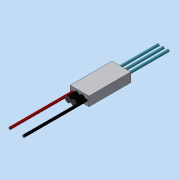
# Autodesk Inventor part: Turnigy_ESC
Saved by Autodesk Inventor 2015 SP1 (Build 190203100, 203)
## iProperties
Created: 2015-06-19
Part Number: Turnigy_ESC
Material: PPS Plastic
Document SubType Name: Modeling
Designer: YOUR_NAME_HERE
Density: 1.637 g/cm^3
Appearance: Smooth - White
Author: YOUR_NAME_HERE
Autodesk Inventor part; units mm, degrees
ref_plane "YZ Plane" through (0, 0, 0) normal (1, 0, 0) x (0, 1, 0)
ref_plane "XZ Plane" through (0, 0, 0) normal (0, 1, 0) x (-1, 0, 0)
ref_plane "XY Plane" through (0, 0, 0) normal (0, 0, 1) x (1, 0, 0)
sketch "Sketch1" plane through (0, 0, 0) normal (0, 1, 0) x (-1, 0, 0)
  line L0 (17, 38) -> (-17, 38)
  line L1 (-17, 38) -> (-17, -38)
  line L2 (-17, -38) -> (17, -38)
  line L3 (17, -38) -> (17, 38)
  line L4 (23.8, 0) -> (-23.8, 0) projected
  line L5 (0, -53.2) -> (0, 53.2) projected
  point P0 (0, 0)
  dimension "d0" = 76
  dimension "d1" = 34
  constraints: 8 end point, 2 parallel, 1 horizontal, 1 perpendicular, 2 other
  measures "d0" distance between parallel lines of L0 L2
  measures "d1" distance between parallel lines of L1 L3
extrude "Extrusion1" add sketch "Sketch1" along normal mid plane 17
sketch "Sketch2" plane through (-17, 8.5, 38) normal (0, 0, 1) x (1, 0, 0)
  line L0 (34, -17) -> (34, 0) projected
  line L1 (0, 0) -> (34, 0) projected
  line L2 (0, 0) -> (0, -17) projected
  line L3 (34, -17) -> (0, -17) projected
  circle A0 centre (11.85, -8.5) radius 5.15
  circle A1 centre (22.15, -8.5) radius 5.15
  line L4 (11.85, -8.5) -> (22.15, -8.5) construction
  circle A2 centre (4.55, -8.5) radius 2.15
  circle A3 centre (29.45, -8.5) radius 2.15
  point P0 (17, -8.5)
  point P1 (17, -8.5)
  dimension "d4" = 10.3
  dimension "d7" = 4.3
  constraints: 4 centre point, 3 tangent, 2 end point, 2 equal radius, 2 point on line, 1 coincident, 1 horizontal, 1 midpoint
  measures "d4" diameter of A1
  measures "d7" diameter of A2
extrude "Extrusion2" add sketch "Sketch2" along normal blind 16 contours A0 | A1
extrude "Extrusion3" add sketch "Sketch2" along normal blind 114.3 contours A2 | A3
sketch "Sketch3" plane through (17, 8.5, -38) normal (0, 0, -1) x (-1, 0, 0)
  circle A0 centre (17, -8.5) radius 2.15
  circle A1 centre (26, -8.5) radius 2.15
  circle A2 centre (8, -8.5) radius 2.15
  dimension "d10" = 4.3
  dimension "d11" = 9
  dimension "d12" = 9
  constraints: 3 centre point, 2 equal radius, 2 horizontal alignment, 1 coincident
  measures "d10" diameter of A1
  measures "d11" distance of point (17, -8.5) A2.centre
  measures "d12" distance of point (17, -8.5) A1.centre
extrude "Extrusion4" add sketch "Sketch3" along normal blind 76.2
body "Solid1"
